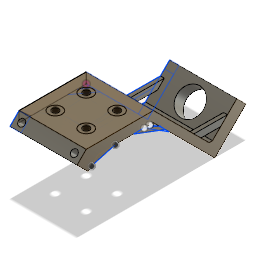
krep (Autodesk Fusion 360 design; units mm, degrees)
Autodesk Fusion 360 part; units mm, degrees
note: some values were not read from the file. Set by a fixed rule: which face or edge a step refers to.
sketch "Sketch1" plane through (0, 0, 0) normal (1, 0, 0) x (0, 0, -1)
  line L0 (0, 0) -> (0, 8)
  line L1 (0, 8) -> (-51, 8)
  line L2 (-51, 8) -> (-51, 0)
  line L3 (-51, 0) -> (0, 0)
  line L4 (-51, 8) -> (-58, 1)
  line L5 (-51, 8) -> (-42.0557, 0)
  line L6 (-58, 1) -> (-51, 8)
  line L7 (-51, 8) -> (-43.2218, 0.2218)
  line L8 (-43.2218, 0.2218) -> (-43.2218, 0)
  line L9 (-58, 1) -> (-49.5147, -7.4853)
  line L10 (-49.5147, -7.4853) -> (-42.0557, 0)
  line L11 (0, 0) -> (46.669, -46.6691)
  line L12 (0, 8) -> (0, 0)
  line L13 (46.669, -46.6691) -> (66.468, -26.8701)
  line L14 (66.468, -26.8701) -> (59.397, -19.799)
  line L15 (59.397, -19.799) -> (39.598, -39.598)
  line L16 (0, 8) -> (50.669, -42.6691)
  line L17 (43.598, -35.598) -> (63.397, -15.799)
  line L18 (63.397, -15.799) -> (70.468, -22.8701)
  line L19 (70.468, -22.8701) -> (46.669, -46.6691)
  line L20 (-14, 0) -> (10.4369, -10.437)
  line L21 (-7, 0) -> (5.2185, -5.2185)
  line L22 (-3.0292, -1.6959) -> (-2.3049, 0)
  line L23 (1.3363, -1.3363) -> (0.533, -3.2173)
  line L24 (30.7391, -22.7391) -> (56.2957, -22.9003)
  line L25 (36.0856, -28.0856) -> (51.1217, -28.0743)
  line L26 (42.2082, -34.2082) -> (44.9129, -34.2831)
  dimension "d1" = 8
  dimension "d2" = 51
  dimension "d3" = 12
  dimension "d4" = 11
  dimension "d5" = 12
  dimension "d6" = 66
  dimension "d7" = 28
  dimension "d8" = 10
  dimension "d9" = 28
  dimension "d10" = 10
  constraint coincident L0.start L3.end
  constraint vertical L0
  constraint perpendicular L0 L1
  constraint perpendicular L1 L2
  constraint perpendicular L0 L3
  constraint coincident L3 L5.end
  constraint parallel L4 L6
  constraint perpendicular L6 L7
  constraint coincident L3 L8.end
  constraint perpendicular L3 L8
  constraint perpendicular L6 L9
  constraint parallel L9 L11
  constraint perpendicular L11 L13
  constraint perpendicular L13 L14
  constraint coincident L11 L15.end
  constraint perpendicular L11 L15
  constraint coincident L13 L16.end
  constraint perpendicular L13 L16
  constraint coincident L16 L17.start
  constraint coincident L15 L17.start
  constraint perpendicular L16 L17
  constraint perpendicular L17 L18
  constraint coincident L3 L20.start
  constraint coincident L11 L20.end
  constraint coincident L3 L21.start
  constraint coincident L11 L21.end
  constraint parallel L20 L21
  constraint coincident L21 L22.start
  constraint coincident L3 L22.end
  constraint perpendicular L21 L22
  constraint coincident L11 L23.start
  constraint coincident L21 L23.end
  constraint perpendicular L21 L23
  constraint coincident L16 L24.start
  constraint coincident L17 L24.end
  constraint coincident L16 L25.start
  constraint coincident L15 L25.end
  constraint coincident L16 L26.start
  constraint coincident L17 L26.end
  measures "d1" distance of L0.start L0.end
  measures "d2" distance of L0.end L1.end
  measures "d3" distance of L1.end L5.end
  measures "d4" distance of L1.end L7.end
  measures "d5" distance of L4.end L9.end
  measures "d6" distance of L0.start L11.end
  measures "d7" distance of L11.end L13.end
  measures "d8" distance of L13.end L14.end
  measures "d9" distance of L17.start L17.end
  measures "d10" distance of L17.end L18.end
extrude "Extrude1" add sketch "Sketch1" along normal blind 51 contours L0 L1 L3 L5 L12 | L3 L11 L21 L22 L23 | L0 L11 L12 L15 L16 | L2 L3 L7 L8 | L2 L3 L4 L6 L9 L10 | L3 L11 L20 L21 | L13 L14 L15 L16 L17 L19 | L15 L16 L17 L26 | L14 L17 L18 L19 | L11 L13 L15 L16 L19 makes body 1
extrude "Extrude2" add sketch "Sketch1" along normal blind 51 and the other way blind -48 separate body contours L15 L16 L17 L24 L25 makes body 2
extrude "Extrude3" add sketch "Sketch1" along normal blind 3 separate body contours L15 L16 L17 L24 L25 makes body 3
extrude "Extrude4" add sketch "Sketch1" along normal blind 51 contours L3 L5 L7 L8 bodies 1
sketch "Sketch2" plane through (0, -39.598, -39.598) normal (0, 0.707107, 0.707107) x (1, 0, 0)
  line L0 (0, 33.6569) -> (0, 7.5164)
  line L1 (0, 7.5164) -> (51, 7.5164)
  line L2 (51, 7.5164) -> (51, 33.6569)
  line L3 (51, 33.6569) -> (0, 33.6569)
  line L4 (0, 33.6569) -> (51, 5.65)
  line L5 (51, 5.65) -> (51, 33.6569)
  line L6 (51, 33.6569) -> (0, 5.65)
  circle A0 centre (25.5, 19.6534) radius 10
  dimension "d21" = 20
  constraint coincident L0.start L3.end
  constraint coincident L2.end L3.start
  constraint midpoint L4 A0.centre
  measures "d21" diameter of A0
extrude "Extrude5" cut sketch "Sketch2" against normal blind 8 contours L4 L6 A0 | L4 L6 A0 | L4 L6 A0 | L4 L6 A0 bodies 1
extrude "Extrude6" cut 1 faces at (28.1433, -31.076, -59.4336) along direction (0, -0.707107, -0.707107) blind 28 on bodies 1 bodies 1
thread "Thread1" "ISO Metric profile 20.0 M20x2.5 6H" major diameter 20.2925 minor diameter 17.519 pitch 2.5 angle 60 resizes the face on face at (35.4876, -31.9481, -60.4472) on face at (35.4503, -28.7681, -57.9703) on bodies 1
sketch "Sketch3" plane through (0, 8, 0) normal (0, 1, 0) x (-1, 0, 0)
  line L0 (0, 0) -> (0, 51)
  line L1 (0, 51) -> (-51, 51)
  line L2 (-51, 51) -> (-51, 0)
  line L3 (-51, 0) -> (0, 0)
  line L4 (-51, 0) -> (-39, 0)
  line L5 (-39, 0) -> (-39, 12)
  line L6 (-39, 12) -> (-51, 12)
  line L7 (-51, 12) -> (-51, 0)
  line L8 (-51, 51) -> (-39, 51)
  line L9 (-39, 51) -> (-39, 39)
  line L10 (-39, 39) -> (-51, 39)
  line L11 (-51, 39) -> (-51, 51)
  line L12 (0, 51) -> (-12, 51)
  line L13 (-12, 51) -> (-12, 39)
  line L14 (-12, 39) -> (0, 39)
  line L15 (0, 39) -> (0, 51)
  line L16 (0, 0) -> (-12, 0)
  line L17 (-12, 0) -> (-12, 12)
  line L18 (-12, 12) -> (0, 12)
  line L19 (0, 12) -> (0, 0)
  circle A0 centre (-13.7943, 13.7408) radius 2.5
  circle A1 centre (-37.2322, 13.7678) radius 2.5
  circle A2 centre (-37.2322, 37.2322) radius 2.5
  circle A3 centre (-13.7678, 37.2322) radius 2.5
  dimension "d26" = 5
  dimension "d27" = 5
  dimension "d28" = 5
  dimension "d29" = 5
  constraint horizontal L4
  constraint vertical L5
  constraint horizontal L6
  constraint vertical L7
  constraint coincident L2.end L3.start
  constraint horizontal L8
  constraint vertical L9
  constraint horizontal L10
  constraint vertical L11
  constraint coincident L1.end L2.start
  constraint horizontal L12
  constraint vertical L13
  constraint horizontal L14
  constraint vertical L15
  constraint coincident L0.end L1.start
  constraint horizontal L16
  constraint vertical L17
  constraint horizontal L18
  constraint vertical L19
  constraint coincident L0.start L3.end
  constraint coincident L17.end A0
  constraint coincident L5.end A1
  constraint coincident L9.end A2
  constraint coincident L13.end A3
  measures "d26" diameter of A0
  measures "d27" diameter of A1
  measures "d28" diameter of A2
  measures "d29" diameter of A3
extrude "Extrude7" cut sketch "Sketch3" against normal blind 37 contours A3 | A2 | A1 | A0 bodies 1
thread "Thread2" "ISO Metric profile 5.0 M5x0.8 6H" major diameter 5.12 minor diameter 4.234 pitch 0.8 angle 60 resizes the face on face at (34.7447, 5.3333, 37.4812) on bodies 1
thread "Thread3" "ISO Metric profile 5.0 M5x0.8 6H" major diameter 5.12 minor diameter 4.234 pitch 0.8 angle 60 resizes the face on face at (39.3037, 2.2044, 12.3682) on bodies 1
thread "Thread4" "ISO Metric profile 5.0 M5x0.8 6H" major diameter 5.12 minor diameter 4.234 pitch 0.8 angle 60 resizes the face on face at (15.8757, 2.203, 12.3559) on bodies 1
thread "Thread5" "ISO Metric profile 5.0 M5x0.8 6H" major diameter 5.12 minor diameter 4.234 pitch 0.8 angle 60 resizes the face on face at (11.2802, 5.3333, 37.4812) on bodies 1
sketch "Sketch4" plane through (0, 8, 0) normal (0, 1, 0) x (-1, 0, 0)
  circle A0 centre (-13.7678, 37.2322) radius 2.117
  circle A1 centre (-37.2322, 13.7678) radius 2.117
  circle A2 centre (-13.7943, 13.7408) radius 2.117
  circle A3 centre (-37.2322, 37.2322) radius 2.117
  line L0 (0, 0) -> (0, 51)
  line L1 (0, 51) -> (-51, 51)
  line L2 (-51, 51) -> (-51, 0)
  line L3 (-51, 0) -> (0, 0)
  circle A4 centre (-13.7678, 37.2322) radius 5
  circle A5 centre (-13.7943, 13.7408) radius 5
  circle A6 centre (-37.2322, 13.7678) radius 5
  circle A7 centre (-37.2322, 37.2322) radius 5
  dimension "d32" = 10
  dimension "d33" = 10
  dimension "d34" = 10
  dimension "d35" = 10
  constraint concentric A0 A4
  constraint concentric A2 A5
  constraint concentric A1 A6
  constraint concentric A3 A7
  measures "d32" diameter of A4
  measures "d33" diameter of A5
  measures "d34" diameter of A6
  measures "d35" diameter of A7
extrude "Extrude8" cut sketch "Sketch4" sketch "Sketch3" along normal blind -3.5 and the other way blind 8 contours A0 | A3 | A4 | A5 | A6 | A7 of sketch 2 contours A1 | A0 bodies 1
extrude "Extrude9" cut sketch "Sketch4" along normal blind -4 and the other way blind 21 contours A5 | A6 bodies 1
extrude "Extrude10" cut sketch "Sketch1" along normal blind 90 contours L3 L11 L20 L21 bodies 1
extrude "Extrude11" cut sketch "Sketch1" along normal blind 85 contours L3 L11 L21 L22 L23 bodies 1
sketch "Sketch5" plane through (0, 29.5, 29.5) normal (0, 0.707107, 0.707107) x (1, 0, 0)
  line L0 (0, -30.4056) -> (0, -40.3051)
  line L1 (0, -40.3051) -> (51, -40.3051)
  line L2 (51, -40.3051) -> (51, -30.4056)
  line L3 (51, -30.4056) -> (0, -30.4056)
  line L4 (0, -35.3553) -> (3, -35.3553)
  line L5 (3, -35.3553) -> (51, -35.3553)
  line L6 (51, -35.3553) -> (48, -35.3553)
  circle A0 centre (5.5, -35.3553) radius 2.5
  circle A1 centre (45.5, -35.3553) radius 2.5
  dimension "d48" = 3
  dimension "d49" = 3
  dimension "d50" = 5
  dimension "d51" = 5
  constraint midpoint L0 L4.start
  constraint perpendicular L0 L4
  constraint midpoint L2 L5.end
  constraint perpendicular L2 L6
  constraint coincident L4.end A0
  constraint coincident L6.end A1
  measures "d48" distance of L4.start L4.end
  measures "d49" distance of L5.end L6.end
  measures "d50" diameter of A0
  measures "d51" diameter of A1
extrude "Extrude12" cut sketch "Sketch5" against normal blind 38 contours L5 A0 | L5 A0 | L5 A1 | L5 A1 bodies 1
thread "Thread6" "ISO Metric profile 5.0 M5x0.8 6H" major diameter 5.12 minor diameter 4.234 pitch 0.8 angle 60 resizes the face on face at (4.0936, 0.2112, 53.1343) on bodies 1
thread "Thread7" "ISO Metric profile 5.0 M5x0.8 6H" major diameter 5.12 minor diameter 4.234 pitch 0.8 angle 60 resizes the face on face at (44.0936, 0.2112, 53.1343) on bodies 1
sketch "Sketch6" plane through (51, 0, 0) normal (1, 0, 0) x (0, 0, -1)
  line L0 (-42.0557, 0) -> (0, 0)
  line L1 (0, 0) -> (46.669, -46.6691)
  line L2 (46.669, -46.6691) -> (70.468, -22.8701)
  line L3 (70.468, -22.8701) -> (63.397, -15.799)
  line L4 (63.397, -15.799) -> (44.9129, -34.2831)
  line L5 (44.9129, -34.2831) -> (42.2082, -34.2082)
  line L6 (42.2082, -34.2082) -> (0, 8)
  line L7 (0, 8) -> (-51, 8)
  line L8 (-51, 8) -> (-58, 1)
  line L9 (-58, 1) -> (-49.5147, -7.4853)
  line L10 (-49.5147, -7.4853) -> (-42.0557, 0)
  line L11 (-47.0422, -5.0041) -> (-29, 0)
  constraint coincident L10 L11.start
  constraint coincident L0 L11.end
extrude "Extrude13" add sketch "Sketch6" along normal blind -51 and the other way blind 49 contours L0 L10 L11 bodies 1
extrude "Extrude14" add sketch "Sketch6" against normal blind 2 contours L0 L10 L11 bodies 1
sketch "Sketch7" plane through (51, 0, 0) normal (1, 0, 0) x (0, 0, -1)
  line L0 (-7, 0) -> (12, -12)
  line L1 (12, -12) -> (5, -5)
  line L2 (5, -5) -> (-2.9167, 0)
  constraint parallel L0 L2
sketch "Sketch8" plane through (51, 0, 0) normal (1, 0, 0) x (0, 0, -1)
  line L0 (-15, 0) -> (9, -9)
  line L1 (9, -9) -> (4.9233, -4.5)
  line L2 (4.9233, -4.5) -> (-7.6424, 0.2121)
  line L3 (-7.6424, 0.2121) -> (-15, 0)
  constraint parallel L0 L2
extrude "Extrude15" add sketch "Sketch8" along normal blind -51 and the other way blind 46 bodies 1
extrude "Extrude16" add sketch "Sketch8" along normal blind -28 and the other way blind 23 bodies 1
extrude "Extrude17" add sketch "Sketch8" against normal blind 5 bodies 1
sketch "Sketch9" plane through (0, -39.598, -39.598) normal (0, 0.707107, 0.707107) x (1, 0, 0)
  circle A0 centre (25.5, 19.6534) radius 8.7595
  line L0 (0, 33.6569) -> (0, 7.5164)
  line L1 (0, 7.5164) -> (51, 7.5164)
  line L2 (51, 7.5164) -> (51, 33.6569)
  line L3 (51, 33.6569) -> (0, 33.6569)
  line L4 (16.7407, 19.5885) -> (15, 19.5885)
  constraint coincident A0 L4.start
  constraint parallel L3 L4
sketch "Sketch10" plane through (0, 29.5, 29.5) normal (0, 0.707107, 0.707107) x (1, 0, 0)
  circle A0 centre (45.5, -35.3553) radius 2.117
  circle A1 centre (5.5, -35.3553) radius 2.117
  line L0 (0, -30.4056) -> (0, -40.3051)
  line L1 (0, -40.3051) -> (51, -40.3051)
  line L2 (51, -40.3051) -> (51, -30.4056)
  line L3 (51, -30.4056) -> (0, -30.4056)
  circle A2 centre (45.5, -35.3553) radius 2.5
  circle A3 centre (5.5, -35.3553) radius 2.5
  dimension "d70" = 5
  dimension "d71" = 5
  constraint concentric A0 A2
  constraint concentric A1 A3
  measures "d70" diameter of A2
  measures "d71" diameter of A3
extrude "Extrude18" cut sketch "Sketch5" against normal blind 34 contours L5 A0 | L5 A0 bodies 1
extrude "Extrude19" cut sketch "Sketch10" against normal blind 32 contours A0 | A2 bodies 1
extrude "Extrude20" cut sketch "Sketch3" against normal blind 43 contours A3 | A2 | A1 | A0 bodies 1
extrude "Extrude21" cut sketch "Sketch9" sketch "Sketch2" against normal blind 25 contours A0 of sketch 2 contours L4 L6 A0 | L4 L6 A0 | L4 L6 A0 | L4 L6 A0 bodies 1
